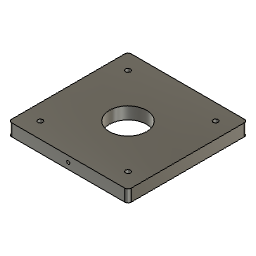
bpod_port_holder (Autodesk Fusion 360 design; units mm, degrees)
Autodesk Fusion 360 part; units mm, degrees
sketch "Sketch1" plane through (0, 0, 0) normal (0, 0, 1) x (1, 0, 0)
  line L0 (0, 0) -> (75, 0)
  line L1 (75, 0) -> (75, 75)
  line L2 (75, 75) -> (0, 75)
  line L3 (0, 75) -> (0, 0)
  circle A0 centre (37.5, 37.5) radius 11.65
  circle A1 centre (10, 65) radius 1.524
  circle A2 centre (65, 65) radius 1.524
  circle A3 centre (10, 10) radius 1.524
  circle A4 centre (65, 10) radius 1.524
  dimension "d1" = 75
  dimension "d2" = 75
  dimension "d3" = 37.5
  dimension "d4" = 37.5
  dimension "d5" = 23.3
  dimension "d6" = 3.048
  dimension "d7" = 10
  dimension "d8" = 10
  dimension "d9" = 10
  dimension "d10" = 10
  dimension "d11" = 10
  dimension "d12" = 10
  dimension "d13" = 10
  dimension "d14" = 10
  constraint horizontal L0
  constraint vertical L1
  constraint horizontal L2
  constraint vertical L3
  constraint coincident L0.start L3.end
  constraint equal A1 A2
  constraint equal A2 A4
  constraint equal A3 A4
  measures "d1" distance of L0 L2
  measures "d2" distance of L1 L3
  measures "d3" distance of L0 A0.centre
  measures "d4" distance of L3 A0.centre
  measures "d5" diameter of A0
  measures "d6" diameter of A1
  measures "d7" distance of L3 A1.centre
  measures "d8" distance of L2 A1.centre
  measures "d9" distance of L2 A2.centre
  measures "d10" distance of L1 A2.centre
  measures "d11" distance of L1 A4.centre
  measures "d12" distance of L0 A4.centre
  measures "d13" distance of L0 A3.centre
  measures "d14" distance of L3 A3.centre
extrude "Extrude1" add sketch "Sketch1" along normal blind 7.62
fillet "Fillet1" radius 2 4 edges at (75, 0, 3.81) (75, 75, 3.81) (0, 0, 3.81) (0, 75, 3.81)
sketch "Sketch2" plane through (0, 0, 0) normal (0, -1, 0) x (1, 0, 0)
  line L0 (2, 7.62) -> (2, 0)
  line L1 (2, 0) -> (73, 0)
  line L2 (73, 0) -> (73, 7.62)
  line L3 (73, 7.62) -> (2, 7.62)
  circle A0 centre (37.5, 3.81) radius 1.016
  dimension "d19" = 35.5
  dimension "d20" = 2.032
  dimension "d21" = 3.81
  measures "d19" distance of L0 A0.centre
  measures "d21" distance of L3 A0.centre
hole "Hole1" at (37.5, 0, 3.81) direction (0, 1, 0) diameter 2.032 depth 30 tip angle 118
